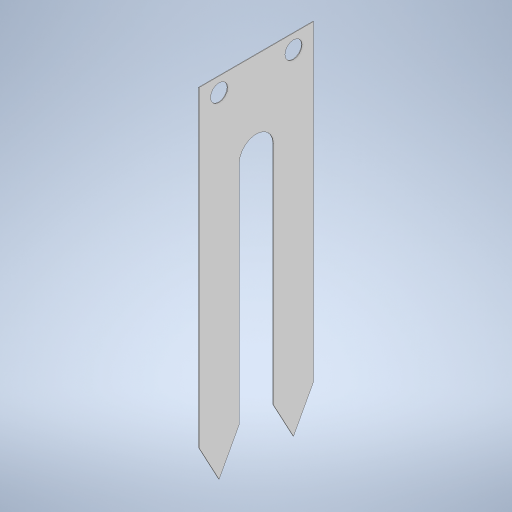
# Autodesk Inventor part: moisture sensor
Saved by Autodesk Inventor 2023 (Build 270158000, 158)
## iProperties
Created: 2023-04-03
Part Number: moisture sensor
Material: Generic
Document SubType Name: Modeling
Designer: user
Density: 1 g/cm^3
Appearance: Default
Author: user
Autodesk Inventor part; units mm, degrees
ref_plane "YZ Plane" through (0, 0, 0) normal (1, 0, 0) x (0, 1, 0)
ref_plane "XZ Plane" through (0, 0, 0) normal (0, 1, 0) x (-1, 0, 0)
ref_plane "XY Plane" through (0, 0, 0) normal (0, 0, 1) x (1, 0, 0)
sketch "Sketch1" plane through (0, 0, 0) normal (1, 0, 0) x (0, 1, 0)
  line L0 (13.5383, 10) -> (13.5383, -10)
  line L1 (13.5383, -10) -> (-40.9617, -10)
  line L2 (-40.9617, -10) -> (-47.4617, -6.5)
  line L3 (-47.4617, -6.5) -> (-40.9617, -3)
  line L4 (-40.9617, -3) -> (-1.4617, -3)
  line L5 (-1.4617, 3) -> (-40.9617, 3)
  line L6 (-40.9617, 3) -> (-47.4617, 6.5)
  line L7 (-47.4617, 6.5) -> (-40.9617, 10)
  line L8 (-40.9617, 10) -> (13.5383, 10)
  arc A0 (-1.4617, -3) -> (-1.4617, 3) centre (-1.4617, 0) ccw
  circle A1 centre (11.0383, 6.5) radius 1.5
  circle A2 centre (11.0383, -6.5) radius 1.5
  point P0 (0, 0)
  point P1 (-13.7117, -10)
  point P2 (13.5383, 10)
  dimension "d0" = 20
  dimension "d1" = 54.5
  dimension "d2" = 7
  dimension "d3" = 7
  dimension "d4" = 6.5
  dimension "d6" = 13.5383
  dimension "d7" = 39.5
  dimension "d8" = 39.5
  dimension "d9" = 3
  dimension "d10" = 6
  dimension "d11" = 10
  dimension "d12" = 61
  dimension "d13" = 1.4617
  dimension "d14" = 54.5
  dimension "d16" = 3
  dimension "d17" = 3.5
  dimension "d19" = 1
  dimension "d20" = 1
  dimension "d21" = 3.5
  dimension "d22" = 3.5
  dimension "d23" = 6.5
  dimension "d24" = 6.5
  dimension "d25" = 3.5
  dimension "d26" = 3.5
  dimension "d27" = 6.5
  dimension "d28" = 3
  dimension "d31" = 6.5
  constraints: 18 end point, 3 centre point, 2 horizontal, 2 point on circle, 1 midpoint, 1 parallel, 1 vertical
  measures "d0" distance of L0.start L0.end
  measures "d1" distance of L0.end L1.end
  measures "d2" distance from line of L4 point (-13.712, -10)
  measures "d3" distance between parallel lines of L8 L5
  measures "d4" horizontal distance of L1.end L2.end
  measures "d6" distance from line of point (0, 0) L0
  measures "d7" distance of L3.end L4.end
  measures "d8" distance of L5.start L5.end
  measures "d9" radius of A0
  measures "d10" distance between parallel lines of L5 L4
  measures "d11" distance from line of L1 point (0, 0)
  measures "d12" distance from line of L2.end L0
  measures "d13" distance of point (0, 0) A0.centre
  measures "d14" distance of L7.end L8.end
  measures "d16" diameter of A2
  measures "d17" distance from line of L8 A1.centre
  measures "d19" distance edge to line of A1 L0
  measures "d20" distance edge to line of A2 L0
  measures "d21" vertical distance of L1.end L2.end
  measures "d22" vertical distance of L2.end L3.end
  measures "d23" horizontal distance of L3.end L2.end
  measures "d24" horizontal distance of L6.end L5.end
  measures "d25" vertical distance of L6.end L5.end
  measures "d26" vertical distance of L7.end L6.end
  measures "d27" horizontal distance of L7.end L6.end
  measures "d28" diameter of A1
  measures "d31" vertical distance of point (0, 0) A2.centre
extrude "Extrusion1" add sketch "Sketch1" along normal blind 0.1
body "Solid1"
